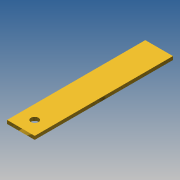
# Autodesk Inventor part: heightMarker
Saved by Autodesk Inventor 2014 SP1 (Build 180222100, 222)
## iProperties
Created: 2014-05-07
Part Number: heightMarker
Material: Gold
Document SubType Name: Modeling
Designer: Dave
Mass: 253.016 g
Surface Area: 110.968 cm^2
Volume: 13.1097 cm^3
Density: 19.3 g/cm^3
Appearance: Gold - Metal
Author: Dave
Autodesk Inventor part; units mm, degrees
ref_plane "YZ Plane" through (0, 0, 0) normal (1, 0, 0) x (0, 1, 0)
ref_plane "XZ Plane" through (0, 0, 0) normal (0, 1, 0) x (-1, 0, 0)
ref_plane "XY Plane" through (0, 0, 0) normal (0, 0, 1) x (1, 0, 0)
sketch "Sketch1" plane through (0, 0, 0) normal (0, 1, 0) x (-1, 0, 0)
  line L0 (0, 0) -> (50.8, 0)
  line L1 (50.8, 0) -> (50.8, 254)
  line L2 (50.8, 254) -> (0, 254)
  line L3 (0, 254) -> (0, 0)
  dimension "d0" = 50.8
  dimension "d1" = 254
  constraints: 8 end point, 2 parallel, 1 horizontal, 1 perpendicular
  measures "d0" distance of L2.end L1.end
  measures "d1" distance of L1.end L0.end
extrude "Extrusion1" add sketch "Sketch1" along normal blind 6.35
sketch "Sketch2" plane through (0, 6.35, 0) normal (0, 1, 0) x (1, 0, 0)
  line L0 (-50.8, -254) -> (0, -254) projected
  circle A0 centre (-25.4, -228.6) radius 6.9766
  dimension "d4" = 25.4
  constraints: 1 centre point
  measures "d4" distance from line of L0 A0.centre
extrude "Extrusion2" cut sketch "Sketch2" against normal blind 25.4
body "Solid1"
